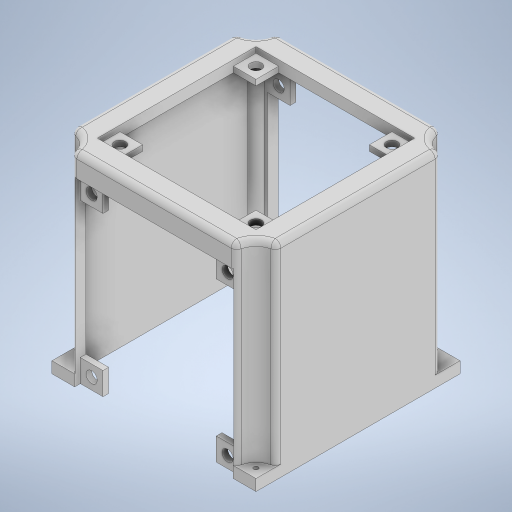
# Autodesk Inventor part: Eg207FinalProjectBox
Saved by Autodesk Inventor 2023 (Build 270158000, 158)
## iProperties
Created: 2023-09-21
Part Number: Eg207FinalProjectBox
Material: Generic
Document SubType Name: Modeling
Designer: Gage
Density: 1 g/cm^3
Appearance: Default
Author: Gage
## iProperties of the stored document Eg207FinalProjectBox_3DPrint.ipt
Created: 2023-09-25
Part Number: Eg207FinalProjectBox_3DPrint
Material: Generic
Document SubType Name: Modeling
Designer: Gage
Density: 1 g/cm^3
Appearance: Default
Author: Gage
Autodesk Inventor part; units mm, degrees
ref_plane "YZ Plane" through (0, 0, 0) normal (1, 0, 0) x (0, 1, 0)
ref_plane "XZ Plane" through (0, 0, 0) normal (0, 1, 0) x (-1, 0, 0)
ref_plane "XY Plane" through (0, 0, 0) normal (0, 0, 1) x (1, 0, 0)
sketch "Sketch1" plane through (0, 0, 0) normal (0, 1, 0) x (-1, 0, 0)
  line L0 (57.15, -57.15) -> (-57.15, -57.15)
  line L1 (-57.15, -57.15) -> (-57.15, 57.15)
  line L2 (-57.15, 57.15) -> (57.15, 57.15)
  line L3 (57.15, 57.15) -> (57.15, -57.15)
  point P0 (0, 0)
  point P1 (-57.15, 0)
  point P2 (0, -57.15)
  dimension "d0" = 114.3
  dimension "d1" = 114.3
  constraints: 8 end point, 2 midpoint, 2 parallel, 1 horizontal, 1 horizontal alignment, 1 perpendicular, 1 vertical alignment
  measures "d0" distance of L1.end L2.end
  measures "d1" distance of L0.end L1.end
extrude "Extrusion1" add sketch "Sketch1" along normal blind 6.35
sketch "Sketch2" plane through (0, 0, 0) normal (0, -1, 0) x (1, 0, 0)
  line L0 (-57.15, 57.15) -> (57.15, 57.15) projected
  line L1 (-57.15, 57.15) -> (57.15, 57.15)
  line L2 (57.15, 57.15) -> (57.15, -57.15)
  line L3 (57.15, -57.15) -> (-57.15, -57.15)
  line L4 (-57.15, -57.15) -> (-57.15, 57.15)
  line L5 (-50.8, 50.8) -> (50.8, 50.8)
  line L6 (50.8, 50.8) -> (50.8, -50.8)
  line L7 (50.8, -50.8) -> (-50.8, -50.8)
  line L8 (-50.8, -50.8) -> (-50.8, 50.8)
  point P0 (0, 0)
  dimension "d4" = 6.35
  dimension "d5" = 6.35
  dimension "d6" = 6.35
  dimension "d7" = 6.35
  constraints: 16 end point, 4 parallel, 2 horizontal, 2 perpendicular
  measures "d4" distance from line of L0 L5.start
  measures "d5" distance from line of L4 L5.start
  measures "d6" distance from line of L2 L6.end
  measures "d7" distance from line of L3 L6.end
extrude "Extrusion2" add sketch "Sketch2" along normal blind 107.95
sketch "Sketch3" plane through (0, 6.35, 0) normal (0, 1, 0) x (1, 0, 0)
  line L0 (-50.8, -50.8) -> (-50.8, 50.8) projected
  line L1 (50.8, 50.8) -> (50.8, -50.8) projected
  line L2 (-50.8, 50.8) -> (50.8, 50.8)
  line L3 (50.8, 50.8) -> (50.8, -50.8)
  line L4 (50.8, -50.8) -> (-50.8, -50.8)
  line L5 (-50.8, -50.8) -> (-50.8, 50.8)
  line L6 (-44.45, 44.45) -> (44.45, 44.45)
  line L7 (44.45, 44.45) -> (44.45, -44.45)
  line L8 (44.45, -44.45) -> (-44.45, -44.45)
  line L9 (-44.45, -44.45) -> (-44.45, 44.45)
  point P0 (0, 0)
  dimension "d10" = 6.35
  dimension "d11" = 6.35
  dimension "d12" = 6.35
  dimension "d13" = 6.35
  constraints: 16 end point, 4 parallel, 2 horizontal, 2 perpendicular
  measures "d10" distance from line of L2 L6.start
  measures "d11" distance from line of L0 L6.start
  measures "d12" distance from line of L1 L7.end
  measures "d13" distance from line of L4 L7.end
extrude "Extrusion3" cut sketch "Sketch3" against normal blind 107.95 contours L6 L7 L8 L9
sketch "Sketch4" plane through (-57.15, 6.35, 57.15) normal (0, 0, 1) x (1, 0, 0)
  line L0 (0, 0) -> (114.3, 0) projected
  line L1 (0, 0) -> (0, -114.3) projected
  line L2 (114.3, -114.3) -> (114.3, 0) projected
  line L3 (114.3, -114.3) -> (0, -114.3) projected
  line L4 (12.7, -12.7) -> (101.6, -12.7)
  line L5 (101.6, -12.7) -> (101.6, -101.6)
  line L6 (101.6, -101.6) -> (12.7, -101.6)
  line L7 (12.7, -101.6) -> (12.7, -12.7)
  line L8 (12.7, -101.6) -> (101.6, -101.6)
  line L9 (101.6, -101.6) -> (101.6, -114.3)
  line L10 (101.6, -114.3) -> (12.7, -114.3)
  line L11 (12.7, -114.3) -> (12.7, -101.6)
  point P0 (57.15, -6.35)
  point P1 (12.7, -114.3)
  dimension "d16" = 12.7
  dimension "d17" = 12.7
  dimension "d18" = 12.7
  dimension "d19" = 12.7
  constraints: 16 end point, 4 parallel, 2 horizontal, 2 perpendicular, 1 point on line
  measures "d16" distance from line of L0 L4.start
  measures "d17" distance from line of L1 L4.start
  measures "d18" distance from line of L2 L5.end
  measures "d19" distance from line of L3 L5.end
extrude "Extrusion4" cut sketch "Sketch4" against normal blind 12.7 contours L11 L6 L9 L3 | L7 L4 L5 L6
ref_plane "Work Plane1" through (0, 0, 0) normal (0, -1, 0) x (1, 0, 0)
sketch "Sketch5" plane through (0, 0, 0) normal (0, -1, 0) x (1, 0, 0)
  line L0 (-44.45, -44.45) -> (44.45, -44.45) projected
  line L1 (-44.45, -44.45) -> (-31.75, -44.45)
  line L2 (-31.75, -44.45) -> (-31.75, -31.75)
  line L3 (-31.75, -31.75) -> (-44.45, -31.75)
  line L4 (-44.45, -31.75) -> (-44.45, -44.45)
  line L5 (44.45, 44.45) -> (44.45, -44.45) projected
  line L6 (44.45, -44.45) -> (31.75, -44.45)
  line L7 (31.75, -44.45) -> (31.75, -31.75)
  line L8 (31.75, -31.75) -> (44.45, -31.75)
  line L9 (44.45, -31.75) -> (44.45, -44.45)
  line L10 (44.45, 44.45) -> (31.75, 44.45)
  line L11 (31.75, 44.45) -> (31.75, 31.75)
  line L12 (31.75, 31.75) -> (44.45, 31.75)
  line L13 (44.45, 31.75) -> (44.45, 44.45)
  line L14 (44.45, 44.45) -> (-44.45, 44.45) projected
  line L15 (-44.45, 44.45) -> (-31.75, 44.45)
  line L16 (-31.75, 44.45) -> (-31.75, 31.75)
  line L17 (-31.75, 31.75) -> (-44.45, 31.75)
  line L18 (-44.45, 31.75) -> (-44.45, 44.45)
  point P0 (0, 0)
  dimension "d23" = 12.7
  dimension "d24" = 12.7
  dimension "d25" = 12.7
  dimension "d26" = 12.7
  dimension "d27" = 12.7
  dimension "d28" = 12.7
  dimension "d29" = 12.7
  dimension "d30" = 12.7
  constraints: 32 end point, 8 parallel, 4 horizontal, 4 perpendicular
  measures "d23" distance of L3.end L2.end
  measures "d24" distance of L2.end L1.end
  measures "d25" distance of L7.end L8.end
  measures "d26" distance of L6.end L7.end
  measures "d27" distance of L12.end L11.end
  measures "d28" distance of L11.end L10.end
  measures "d29" distance of L16.end L17.end
  measures "d30" distance of L15.end L16.end
extrude "Extrusion5" add sketch "Sketch5" against normal blind 3.175
ref_plane "Work Plane2" through (50.8, 0, 50.8) normal (0, 0, -1) x (-1, 0, 0)
sketch "Sketch6" plane through (50.8, 0, 50.8) normal (0, 0, -1) x (-1, 0, 0)
  line L0 (6.35, -6.35) -> (95.25, -6.35) projected
  line L1 (95.25, -6.35) -> (82.55, -6.35)
  line L2 (82.55, -6.35) -> (82.55, -19.05)
  line L3 (82.55, -19.05) -> (95.25, -19.05)
  line L4 (95.25, -19.05) -> (95.25, -6.35)
  line L5 (6.35, -107.95) -> (6.35, -6.35) projected
  line L6 (6.35, -6.35) -> (19.05, -6.35)
  line L7 (19.05, -6.35) -> (19.05, -19.05)
  line L8 (19.05, -19.05) -> (6.35, -19.05)
  line L9 (6.35, -19.05) -> (6.35, -6.35)
  line L10 (95.25, -6.35) -> (95.25, -107.95) projected
  line L11 (95.25, -107.95) -> (82.55, -107.95)
  line L12 (82.55, -107.95) -> (82.55, -95.25)
  line L13 (82.55, -95.25) -> (95.25, -95.25)
  line L14 (95.25, -95.25) -> (95.25, -107.95)
  line L15 (0, -107.95) -> (101.6, -107.95) projected
  line L16 (6.35, -107.95) -> (19.05, -107.95)
  line L17 (19.05, -107.95) -> (19.05, -95.25)
  line L18 (19.05, -95.25) -> (6.35, -95.25)
  line L19 (6.35, -95.25) -> (6.35, -107.95)
  point P0 (50.8, 0)
  point P1 (6.35, -95.25)
  dimension "d34" = 12.7
  dimension "d35" = 12.7
  dimension "d36" = 12.7
  dimension "d37" = 12.7
  dimension "d38" = 12.7
  dimension "d39" = 12.7
  dimension "d40" = 12.7
  dimension "d41" = 12.7
  constraints: 32 end point, 8 parallel, 4 horizontal, 4 perpendicular, 2 point on line
  measures "d34" distance of L3.end L2.end
  measures "d35" distance of L2.end L1.end
  measures "d36" distance of L7.end L8.end
  measures "d37" distance of L6.end L7.end
  measures "d38" distance of L12.end L13.end
  measures "d39" distance of L11.end L12.end
  measures "d40" distance of L18.end L17.end
  measures "d41" distance of L17.end L16.end
extrude "Extrusion6" add sketch "Sketch6" against normal blind 3.175 contours L0 L7 L8 L5 | L0 L4 L3 L2 | L18 L17 L15 L5 | L10 L11 L12 L13
sketch "Sketch7" plane through (0, 3.175, 0) normal (0, 1, 0) x (1, 0, 0)
  circle A0 centre (38.1, 38.1) radius 3.175
  circle A1 centre (-38.1, 38.1) radius 3.175
  circle A2 centre (-38.1, -38.1) radius 3.175
  circle A3 centre (38.1, -38.1) radius 3.175
  line L0 (-44.45, 44.45) -> (44.45, 44.45) projected
  line L1 (-44.45, -44.45) -> (-44.45, 44.45) projected
  line L2 (44.45, 44.45) -> (44.45, -44.45) projected
  line L3 (44.45, -44.45) -> (-44.45, -44.45) projected
  line L4 (-31.75, -31.75) -> (-44.45, -31.75) projected
  point P0 (0, 0)
  point P1 (-38.1, -31.75)
  dimension "d44" = 6.35
  dimension "d45" = 6.35
  dimension "d46" = 6.35
  dimension "d47" = 6.35
  dimension "d48" = 6.35
  dimension "d49" = 6.35
  dimension "d50" = 6.35
  dimension "d51" = 6.35
  dimension "d52" = 6.35
  dimension "d53" = 6.35
  dimension "d54" = 6.35
  dimension "d55" = 6.35
  constraints: 4 centre point, 1 midpoint
  measures "d44" diameter of A0
  measures "d45" diameter of A1
  measures "d46" diameter of A2
  measures "d47" diameter of A3
  measures "d48" distance from line of L0 A1.centre
  measures "d49" distance from line of L1 A1.centre
  measures "d50" distance from line of L0 A0.centre
  measures "d51" distance from line of L2 A0.centre
  measures "d52" distance from line of L2 A3.centre
  measures "d53" distance from line of L3 A3.centre
  measures "d54" distance from line of L1 A2.centre
  measures "d55" distance of point (-38.1, -31.75) A2.centre
extrude "Extrusion7" cut sketch "Sketch7" against normal blind 3.175 contours A0 | A1 | A2 | A3
sketch "Sketch8" plane through (50.8, 0, 53.975) normal (0, 0, 1) x (1, 0, 0)
  circle A0 centre (-88.9, -12.7) radius 3.175
  line L0 (-95.25, -6.35) -> (-6.35, -6.35) projected
  line L1 (-95.25, -107.95) -> (-95.25, -6.35) projected
  circle A1 centre (-12.7, -12.7) radius 3.175
  line L2 (-6.35, -6.35) -> (-6.35, -107.95) projected
  circle A2 centre (-12.7, -101.6) radius 3.175
  circle A3 centre (-88.9, -101.6) radius 3.175
  line L3 (-95.25, -107.95) -> (-82.55, -107.95) projected
  line L4 (-19.05, -107.95) -> (-6.35, -107.95) projected
  point P0 (-50.8, 0)
  dimension "d58" = 6.35
  dimension "d59" = 6.35
  dimension "d60" = 6.35
  dimension "d61" = 6.35
  dimension "d62" = 6.35
  dimension "d63" = 6.35
  dimension "d64" = 6.35
  dimension "d65" = 6.35
  dimension "d66" = 6.35
  dimension "d67" = 6.35
  dimension "d68" = 6.35
  dimension "d69" = 6.35
  constraints: 4 centre point
  measures "d58" diameter of A0
  measures "d59" distance from line of L0 A0.centre
  measures "d60" distance from line of L1 A0.centre
  measures "d61" diameter of A1
  measures "d62" distance from line of L0 A1.centre
  measures "d63" distance from line of L2 A1.centre
  measures "d64" diameter of A2
  measures "d65" diameter of A3
  measures "d66" distance from line of L1 A3.centre
  measures "d67" distance from line of L3 A3.centre
  measures "d68" distance from line of L2 A2.centre
  measures "d69" distance from line of L4 A2.centre
extrude "Extrusion8" cut sketch "Sketch8" against normal blind 3.175
sketch "Sketch10" plane through (0, -107.95, 0) normal (0, -1, 0) x (1, 0, 0)
  line L0 (57.15, 57.15) -> (44.45, 57.15) projected
  circle A0 centre (57.15, 57.15) radius 12.7
  line L1 (-57.15, -57.15) -> (57.15, -57.15) projected
  circle A1 centre (57.15, -57.15) radius 12.7
  line L2 (-57.15, 57.15) -> (57.15, 57.15) projected
  circle A2 centre (-57.15, 57.15) radius 12.7
  circle A3 centre (-57.15, -57.15) radius 12.7
  line L3 (50.8, 50.8) -> (-50.8, 50.8) projected
  line L4 (-46.1515, 50.8) -> (-50.8, 50.8)
  line L5 (-50.8, 50.8) -> (-50.8, 46.1515)
  line L6 (-50.8, -50.8) -> (-50.8, 50.8) projected
  line L7 (50.8, 50.8) -> (50.8, 46.1515)
  line L8 (50.8, 50.8) -> (50.8, -50.8) projected
  line L9 (31.75, 50.8) -> (50.8, 50.8) projected
  line L10 (46.1515, 50.8) -> (50.8, 50.8)
  line L11 (50.8, -50.8) -> (50.8, -46.1515)
  line L12 (50.8, -50.8) -> (-50.8, -50.8) projected
  line L13 (50.8, -50.8) -> (46.1515, -50.8)
  line L14 (-50.8, -50.8) -> (-50.8, -46.1515)
  line L15 (-50.8, -50.8) -> (-46.1515, -50.8)
  point P0 (0, 0)
  point P1 (46.1515, 50.8)
  dimension "d72" = 25.4
  dimension "d73" = 25.4
  dimension "d74" = 25.4
  dimension "d75" = 25.4
  constraints: 16 end point, 9 point on line, 8 point on circle, 4 centre point, 2 collinear, 1 coincident
  measures "d72" diameter of A0
  measures "d73" diameter of A1
  measures "d74" diameter of A2
  measures "d75" diameter of A3
extrude "Extrusion9" add sketch "Sketch10" against normal blind 107.95 contours A0 L3 L7 | L8 L12 A1 | L5 L3 A2 | A3 L12 L6 picked at (50.1955, 48.1242) picked at (48.1242, -50.1955) picked at (-50.1955, 48.1242) picked at (-48.1242, -50.1955)
sketch "Sketch11" plane through (0, 6.35, 0) normal (0, 1, 0) x (1, 0, 0)
  circle A0 centre (-57.15, 57.15) radius 11.1125
  line L0 (57.15, 57.15) -> (57.15, -57.15) projected
  circle A1 centre (57.15, 57.15) radius 11.1125
  line L1 (57.15, -57.15) -> (44.45, -57.15) projected
  circle A2 centre (57.15, -57.15) radius 11.1125
  circle A3 centre (-57.15, -57.15) radius 11.1125
  point P0 (0, 0)
  dimension "d78" = 22.225
  dimension "d79" = 22.225
  dimension "d80" = 22.225
  dimension "d81" = 22.225
  constraints: 4 centre point, 1 coincident
  measures "d78" diameter of A0
  measures "d79" diameter of A1
  measures "d80" diameter of A2
  measures "d81" diameter of A3
extrude "Extrusion10" cut sketch "Sketch11" against normal blind 107.95
fillet "Fillet1" radius 3.175 16 edges at (0, 6.35, 57.15) (57.15, 6.35, 0) (0, 6.35, -57.15) (-57.15, 6.35, 0) (57.15, -47.625, 46.0375) (46.0375, -47.625, 57.15) (-46.0375, -47.625, 57.15) (-57.15, -47.625, 46.0375) (57.15, -47.625, -46.0375) (46.0375, -47.625, -57.15) (-46.0375, -47.625, -57.15) (-57.15, -47.625, -46.0375) (-49.2923, 6.35, -49.2923) (49.2923, 6.35, -49.2923) (49.2923, 6.35, 49.2923) (-49.2923, 6.35, 49.2923)
sketch "Sketch12" plane through (0, -101.6, 0) normal (0, 1, 0) x (1, 0, 0)
  circle A0 centre (52.07, -52.07) radius 3.5498
  line L0 (57.15, -43.2197) -> (57.15, -57.15) projected
  line L1 (44.45, -57.15) -> (57.15, -57.15) projected
  point P0 (0, 0)
  dimension "d85" = 5.08
  dimension "d86" = 5.08
  constraints: 1 centre point
  measures "d85" distance from line of L0 A0.centre
  measures "d86" distance from line of L1 A0.centre
hole "Hole1" at (52.07, -101.6, 52.07) direction (0, -1, 0) diameter 2.6416 end through all start extended yes thread size "6-32 UNC" class "2B" standard "ANSI Unified Screw Threads"
mirror "Mirror1" about plane through (0, 0, 0) normal (0, 0, 1) of "Extrusion4"
mirror "Mirror2" about plane through (0, 0, 0) normal (0, 0, 1) of "Extrusion6"
mirror "Mirror3" about plane through (0, 0, 0) normal (0, 0, 1) of "Extrusion8"
body "Solid1"
